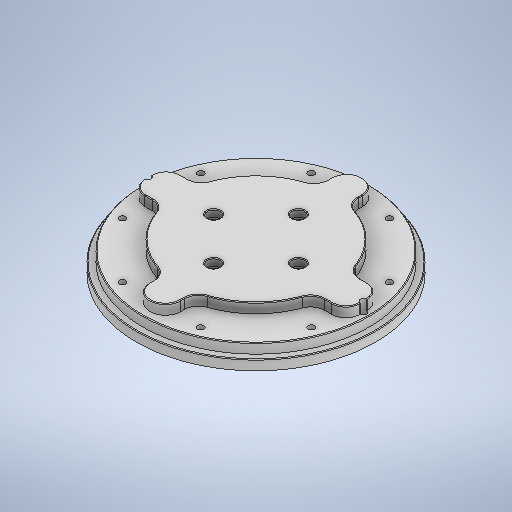
# Autodesk Inventor part: Updated Build Platform
Saved by Autodesk Inventor 2025 (Build 290162000, 162)
## iProperties
Created: 2025-09-30
Part Number: Updated Build Platform
Material: Generic
Document SubType Name: Modeling
Designer: mumin
Density: 1 g/cm^3
Appearance: Default
Author: mumin
Autodesk Inventor part; units mm, degrees
ref_plane "YZ Plane" through (0, 0, 0) normal (1, 0, 0) x (0, 1, 0)
ref_plane "XZ Plane" through (0, 0, 0) normal (0, 1, 0) x (-1, 0, 0)
ref_plane "XY Plane" through (0, 0, 0) normal (0, 0, 1) x (1, 0, 0)
sketch "Sketch1" plane through (0, 0, 0) normal (1, 0, 0) x (0, 1, 0)
  line L0 (0, 0) -> (14, 0)
  line L1 (14, 0) -> (14, -79.5)
  line L2 (13.5, -80) -> (7, -80)
  line L3 (7, -80) -> (7, -84)
  line L4 (6.5, -84.5) -> (0, -84.5)
  line L5 (0, -84.5) -> (0, 0)
  line L6 (0, 0) -> (14, 0)
  line L7 (14, -79.5) -> (13.5, -80)
  line L8 (7, -84) -> (6.5, -84.5)
  point P0 (14, -80)
  point P1 (7, -84.5)
  dimension "d1" = 80
  dimension "d2" = 84.5
  dimension "d3" = 7
  dimension "d4" = 7
  dimension "d5" = 0.5
  dimension "d6" = 0.5
  dimension "d7" = 0.5
  dimension "d8" = 0.5
  constraints: 18 end point, 5 point on line, 4 perpendicular, 1 horizontal, 1 parallel, 1 vertical
  measures "d1" distance between parallel lines of L6 L2
  measures "d2" distance between parallel lines of L6 L4
  measures "d3" distance of point (14, -80) L2.end
  measures "d4" distance of point (7, -84.5) L4.end
  measures "d5" distance of L1.end point (14, -80)
  measures "d6" distance of L2.start point (14, -80)
  measures "d7" distance of L3.end point (7, -84.5)
  measures "d8" distance of L4.start point (7, -84.5)
revolve "Base" add sketch "Sketch1" angle 360 about axis through (0, 0, 0) along (0, 1, 0)
sketch "Sketch2" plane through (0, 14, 0) normal (0, 1, 0) x (1, 0, 0)
  circle A0 centre (0, 0) radius 55
  line L0 (0, 118.3) -> (0, -118.3)
  line L1 (-76, -2.5) -> (-76, 2.5)
  arc A1 (-76, -2.5) -> (-66, -12.5) centre (-66, -2.5) ccw
  line L2 (-66, -2.5) -> (-66, -12.5) construction
  line L3 (-66, -2.5) -> (-76, -2.5) construction
  arc A2 (-66, 12.5) -> (-76, 2.5) centre (-66, 2.5) ccw
  line L4 (-118.3, 0) -> (118.3, 0)
  line L5 (-66, -12.5) -> (-60.981555, -12.5)
  line L6 (-66, 12.5) -> (-60.981555, 12.5)
  arc A3 (-60.981555, 12.5) -> (-51.599777, 19.038462) centre (-60.981555, 22.5) ccw
  arc A4 (-51.599777, -19.038462) -> (-60.981555, -12.5) centre (-60.981555, -22.5) ccw
  line L7 (76, -2.5) -> (76, 2.5)
  arc A5 (66, -12.5) -> (76, -2.5) centre (66, -2.5) ccw
  line L8 (66, -2.5) -> (66, -12.5) construction
  line L9 (66, -2.5) -> (76, -2.5) construction
  arc A6 (76, 2.5) -> (66, 12.5) centre (66, 2.5) ccw
  line L10 (66, -12.5) -> (60.981555, -12.5)
  line L11 (66, 12.5) -> (60.981555, 12.5)
  arc A7 (51.599777, 19.038462) -> (60.981555, 12.5) centre (60.981555, 22.5) ccw
  arc A8 (60.981555, -12.5) -> (51.599777, -19.038462) centre (60.981555, -22.5) ccw
  line L12 (-10.9, -64.1) -> (-10.9, -61.548274)
  arc A9 (-10.9, -61.548274) -> (-17.684615, -52.079309) centre (-20.9, -61.548274) ccw
  line L13 (10.9, -64.1) -> (10.9, -61.548274)
  arc A10 (17.684615, -52.079309) -> (10.9, -61.548274) centre (20.9, -61.548274) ccw
  arc A11 (-10.9, -64.1) -> (10.9, -64.1) centre (0, -64.1) ccw
  line L14 (-10.9, 64.1) -> (-10.9, 61.548274)
  arc A12 (-17.684615, 52.079309) -> (-10.9, 61.548274) centre (-20.9, 61.548274) ccw
  arc A13 (10.9, 61.548274) -> (17.684615, 52.079309) centre (20.9, 61.548274) ccw
  line L15 (10.9, 64.1) -> (10.9, 61.548274)
  arc A14 (10.9, 64.1) -> (-10.9, 64.1) centre (0, 64.1) ccw
  dimension "d10" = 110
  dimension "d14" = 90
  dimension "d15" = 10
  dimension "d16" = 25
  dimension "d17" = 76
  dimension "d19" = 10
  dimension "d22" = 64.1
  dimension "d23" = 10
  constraints: 30 point on circle, 29 symmetric about line, 28 end point, 15 centre point, 7 tangent, 2 horizontal, 2 vertical, 1 coincident, 1 point on line, 9 other
  measures "d10" diameter of A0
  measures "d14" angle of L3 L2
  measures "d15" radius of A1
  measures "d16" distance of L6.start L2.end
  measures "d17" distance from line of point (0, 0) L1
  measures "d19" radius of A3
  measures "d22" distance of point (0, 0) A11.centre
  measures "d23" radius of A9
extrude "Clover" add sketch "Sketch2" along normal blind 7
sketch "Sketch3" plane through (0, 21, 0) normal (0, 1, 0) x (1, 0, 0)
  circle A0 centre (0, 0) radius 29.95 construction
  line L0 (-118.3, 0) -> (118.3, 0) construction
  point P0 (-29.95, 0)
  dimension "d33" = 59.9
  constraints: 1 coincident, 1 horizontal alignment, 1 point on line, 2 other
hole "Plunger Mount Holes" at (-29.95, 21, 0) direction (0, -1, 0) diameter 5.5 end through all counterbore diameter 9 counterbore depth 5
pattern_circular "Circular Pattern1" count 4 over 360 about axis through (0, -10, 0) along (0, 1, 0) of "Plunger Mount Holes"
sketch "Sketch4" plane through (0, 14, 0) normal (0, 1, 0) x (1, 0, 0)
  circle A0 centre (0, 0) radius 72.25 construction
  line L0 (0, 0) -> (-66.750296, 27.648878) construction
  line L1 (-118.3, 0) -> (118.3, 0) construction
  point P0 (-66.750296, 27.648878)
  dimension "d45" = 144.5
  dimension "d46" = 22.5
  constraints: 2 coincident, 2 end point, 3 other
  measures "d46" angle of L1 L0
hole "Seal Ring Holes" at (-66.750296, 14, -27.648878) direction (0, -1, 0) diameter 4.4 end through all
pattern_circular "Circular Pattern2" count 8 over 360 about axis through (0, -10, 0) along (0, 1, 0) of "Seal Ring Holes"
sketch "Sketch5" plane through (0, 21, 0) normal (0, 1, 0) x (1, 0, 0)
  line L0 (-76, 2.5) -> (-76, -2.5) projected
  point P0 (0, 0)
  point P1 (-76, 0)
  point P2 (-76, 0)
  constraints: 1 coincident, 1 midpoint
hole "Plate Mounting Holes" at (-76, 21, 0) direction (0, -1, 0) diameter 4.4 end through all
mirror "Mirror1" about plane through (0, 0, 0) normal (1, 0, 0) of "Plate Mounting Holes"
sketch "Sketch6" plane through (0, 0, 0) normal (0, -1, 0) x (1, 0, 0)
  circle A0 centre (0, 0) radius 40
  line L0 (35, 19.364917) -> (35, -19.364917)
  dimension "d57" = 80
  dimension "d58" = 35
  constraints: 2 end point, 2 point on circle, 1 centre point, 1 coincident, 1 vertical
  measures "d57" diameter of A0
  measures "d58" distance from line of L0 point (0, 0)
extrude "Key Shape" cut sketch "Sketch6" against normal blind 1.5 contours L0 A0 picked at (4.779497, -0.943376)
sketch "Sketch7" plane through (0, 1.5, 0) normal (0, -1, 0) x (1, 0, 0)
  circle A0 centre (0, 0) radius 10
  dimension "d61" = 20
  constraints: 1 centre point, 1 coincident
  measures "d61" diameter of A0
extrude "Bolt Recess" cut sketch "Sketch7" against normal blind 6
chamfer "Chamfer1" distance 0.5 angle 45 34 edges at (-73.0711, 21, 9.5711) (-63.4908, 21, 12.5) (-55.2638, 21, 14.2959) (-38.3798, 21, 39.3954) (-12.7712, 21, 55.7239) (-10.9, 21, 62.8241) (0, 21, 75) (10.9, 21, 62.8241) (12.7712, 21, 55.7239) (38.3798, 21, 39.3954) (55.2638, 21, 14.2959) (63.4908, 21, 12.5) (73.0711, 21, 9.5711) (76, 21, 2.35) (-76, 21, 2.35) (-63.4908, 21, -12.5) (-73.0711, 21, -9.5711) (-76, 21, -2.35) (-55.2638, 21, -14.2959) (-38.3798, 21, -39.3954) (-12.7712, 21, -55.7239) (-10.9, 21, -62.8241) (0, 21, -75) (10.9, 21, -62.8241) (12.7712, 21, -55.7239) (38.3798, 21, -39.3954) (55.2638, 21, -14.2959) (63.4908, 21, -12.5) (73.0711, 21, -9.5711) (76, 21, -2.35) (-29.95, 21, -4.5) (4.5, 21, -29.95) (29.95, 21, 4.5) (-4.5, 21, 29.95)
equation "\"d6\" = d5"
equation "\"d7\" = d5"
equation "\"d8\" = d7"
body "Solid1"
